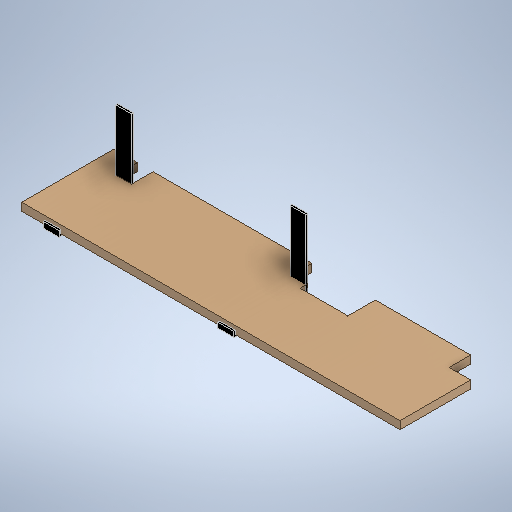
# Autodesk Inventor part: BottomShelf
Saved by Autodesk Inventor 2025 (Build 290162010, 162A)
## iProperties
Created: 2024-08-20
Part Number: BottomShelf
Material: Generic
Document SubType Name: Modeling
Designer: max_d
Density: 1 g/cm^3
Appearance: Default
Author: max_d
Autodesk Inventor part; units mm, degrees
ref_plane "YZ Plane" through (0, 0, 0) normal (1, 0, 0) x (0, 1, 0)
ref_plane "XZ Plane" through (0, 0, 0) normal (0, 1, 0) x (-1, 0, 0)
sketch "Sketch1" plane through (0, 0, 0) normal (1, 0, 0) x (0, 1, 0)
  line L0 (0, 0) -> (0, 190)
  line L1 (0, 190) -> (15, 190)
  line L2 (15, 190) -> (15, 185)
  line L3 (15, 185) -> (5, 185)
  line L4 (5, 185) -> (5, 5)
  line L5 (5, 5) -> (180, 5)
  line L6 (180, 5) -> (180, 0)
  line L7 (180, 0) -> (0, 0)
  line L8 (5, 95) -> (0, 95) construction
  dimension "d0" = 190
  dimension "d1" = 15
  dimension "d2" = 180
  dimension "d3" = 5
  constraints: 18 end point, 10 perpendicular, 2 midpoint, 1 vertical
  measures "d0" distance of L0.start L0.end
  measures "d1" distance of L0.end L1.end
  measures "d2" distance of L6.end L0.start
  measures "d3" distance of L8.start L8.end
extrude "Extrusion1" add sketch "Sketch1" along normal blind 40
fillet "Fillet1" radius 2 2 edges at (20, 0, 190) (20, 0, 0)
sketch "Sketch2" plane through (0, 5, 185) normal (0, 1, 0) x (1, 0, 0)
  line L0 (460, 0) -> (-505, 0)
  line L1 (-505, 0) -> (-505, 235)
  line L2 (-505, 235) -> (460, 235)
  line L3 (460, 235) -> (460, 0)
  line L4 (0, 0) -> (40, 0) projected
  line L5 (40, 180) -> (40, 0) projected
  line L6 (-405, 235) -> (-405, 0) construction
  line L7 (0, 180) -> (0, 0) construction
  line L8 (-445, 235) -> (-445, 0) construction
  line L9 (-445, 180) -> (-405, 180)
  line L10 (-445, 235) -> (-445, 180)
  line L11 (-405, 180) -> (-405, 235)
  line L12 (0, 185) -> (40, 185)
  line L13 (0, 180) -> (40, 180) projected
  line L14 (0, 180) -> (40, 180)
  line L15 (40, 180) -> (40, 235)
  line L16 (0, 180) -> (0, 235)
  line L17 (405, 235) -> (405, 180)
  line L18 (405, 180) -> (460, 180)
  dimension "d8" = 420
  dimension "d9" = 405
  dimension "d10" = 40
  dimension "d11" = 60
  dimension "d14" = 50
  dimension "d15" = 55
  dimension "d16" = 55
  constraints: 30 end point, 10 point on line, 7 perpendicular, 5 collinear, 2 parallel, 1 horizontal, 1 vertical
  measures "d8" distance between parallel lines of L3 L5
  measures "d9" distance between parallel lines of L7 L6
  measures "d10" distance between parallel lines of L6 L8
  measures "d11" distance between parallel lines of L1 L8
  measures "d14" distance between parallel lines of L2 L12
  measures "d15" distance of L17.start L17.end
  measures "d16" distance of L17.end L18.end
extrude "Extrusion2" add sketch "Sketch2" along normal blind 20 separate body contours L0 L5 L15 L2 L17 L18 L3 | L0 L1 L2 L10 L9 L11 L16 L13 L5 | L13 L16 L12 L15
ref_plane "Work Plane1" through (-202.5, 5, -50) normal (-1, 0, 0) x (0, 0, 1)
mirror "Mirror1" about plane through (-202.5, 5, -50) normal (-1, 0, 0) of "Extrusion1" bodies 1
sketch "Sketch3" plane through (-227.623, 25, 187.9845) normal (0, 1, 0) x (1, 0, 0)
  line L0 (267.623, 182.9845) -> (267.623, 2.9845) projected
  line L1 (267.623, 182.9845) -> (267.623, 167.9845)
  line L2 (267.623, 167.9845) -> (389.623, 167.9845)
  line L3 (389.623, 167.9845) -> (389.623, 237.9845)
  line L4 (632.623, 237.9845) -> (267.623, 237.9845) projected
  line L5 (267.623, 237.9845) -> (267.623, 182.9845)
  line L6 (267.623, 237.9845) -> (389.623, 237.9845)
  dimension "d22" = 15
  dimension "d23" = 122
  constraints: 10 end point, 3 perpendicular, 2 point on line, 1 parallel
  measures "d22" distance of L0.start L1.end
  measures "d23" distance of L1.end L2.end
extrude "Extrusion3" cut sketch "Sketch3" against normal blind 20 bodies 2
body "Solid1"
body "Solid2"
